Autodesk Fusion 360 part; units mm, degrees
(part 32 of 40)
  line L7913 (276.237, 134.1758) -> (276.3666, 134.08) construction
  line L7914 (276.3666, 134.08) -> (276.4958, 133.9832) construction
  line L7915 (276.4958, 133.9832) -> (276.6246, 133.8854) construction
  line L7916 (276.6246, 133.8854) -> (276.7529, 133.7868) construction
  line L7917 (276.7529, 133.7868) -> (276.8808, 133.6873) construction
  line L7918 (276.8808, 133.6873) -> (277.0082, 133.5869) construction
  line L7919 (277.0082, 133.5869) -> (277.1352, 133.4856) construction
  line L7920 (277.1352, 133.4856) -> (277.2618, 133.3834) construction
  line L7921 (277.2618, 133.3834) -> (277.388, 133.2804) construction
  line L7922 (277.388, 133.2804) -> (277.5137, 133.1765) construction
  line L7923 (277.5137, 133.1765) -> (277.639, 133.0717) construction
  line L7924 (277.639, 133.0717) -> (277.7638, 132.9662) construction
  line L7925 (277.7638, 132.9662) -> (277.8882, 132.8598) construction
  line L7926 (277.8882, 132.8598) -> (278.0122, 132.7526) construction
  line L7927 (278.0122, 132.7526) -> (278.1358, 132.6445) construction
  line L7928 (278.1358, 132.6445) -> (278.2589, 132.5357) construction
  line L7929 (278.2589, 132.5357) -> (278.3817, 132.4261) construction
  line L7930 (278.3817, 132.4261) -> (278.5039, 132.3158) construction
  line L7931 (278.5039, 132.3158) -> (278.6258, 132.2046) construction
  line L7932 (278.6258, 132.2046) -> (278.7472, 132.0927) construction
  line L7933 (278.7472, 132.0927) -> (278.8682, 131.98) construction
  line L7934 (278.8682, 131.98) -> (278.9888, 131.8665) construction
  line L7935 (278.9888, 131.8665) -> (279.1089, 131.7523) construction
  line L7936 (279.1089, 131.7523) -> (279.2286, 131.6374) construction
  line L7937 (279.2286, 131.6374) -> (279.3479, 131.5218) construction
  line L7938 (279.3479, 131.5218) -> (279.4667, 131.4054) construction
  line L7939 (279.4667, 131.4054) -> (279.5851, 131.2882) construction
  line L7940 (279.5851, 131.2882) -> (279.7031, 131.1704) construction
  line L7941 (279.7031, 131.1704) -> (279.8207, 131.0519) construction
  line L7942 (279.8207, 131.0519) -> (279.9378, 130.9326) construction
  line L7943 (279.9378, 130.9326) -> (280.0545, 130.8127) construction
  line L7944 (280.0545, 130.8127) -> (280.1708, 130.6921) construction
  line L7945 (280.1708, 130.6921) -> (280.2866, 130.5707) construction
  line L7946 (280.2866, 130.5707) -> (280.402, 130.4488) construction
  line L7947 (280.402, 130.4488) -> (280.517, 130.3261) construction
  line L7948 (280.517, 130.3261) -> (280.6087, 130.2274) construction
  line L7949 (280.6087, 130.2274) -> (280.6772, 130.1531) construction
  line L7950 (280.6772, 130.1531) -> (280.7228, 130.1034) construction
  line L7951 (280.7228, 130.1034) -> (280.7456, 130.0785) construction
  spline S106 degree 5 poles (187.9372, 206.0345) (187.9249, 206.0628) (187.9012, 206.1198) (187.868, 206.2062) (187.8281, 206.3229) (187.7842, 206.4711) (187.7447, 206.6208) (187.7079, 206.7714) (187.6725, 206.9226) (187.638, 207.0741) (187.6046, 207.226) (187.5726, 207.3783) (187.5424, 207.5312) (187.5144, 207.6848) (187.4885, 207.8391) (187.4646, 207.994) (187.4423, 208.1494) (187.4215, 208.3052) (187.4019, 208.4614) (187.3835, 208.6179) (187.3662, 208.7747) (187.3502, 208.9318) (187.3355, 209.0893) (187.3222, 209.2471) (187.3102, 209.4053) (187.2995, 209.5638) (187.29, 209.7226) (187.2816, 209.8817) (187.2743, 210.0411) (187.2682, 210.2007) (187.2631, 210.3605) (187.2591, 210.5206) (187.2563, 210.6809) (187.2544, 210.8415) (187.2537, 211.0023) (187.254, 211.1633) (187.2554, 211.3245) (187.2578, 211.4859) (187.2612, 211.6475) (187.2655, 211.8093) (187.2709, 211.9712) (187.2772, 212.1334) (187.2845, 212.2957) (187.2928, 212.4581) (187.302, 212.6207) (187.3121, 212.7835) (187.3232, 212.9464) (187.3353, 213.1095) (187.3482, 213.2727) (187.362, 213.436) (187.3768, 213.5995) (187.3924, 213.7631) (187.409, 213.9268) (187.4264, 214.0906) (187.4447, 214.2545) (187.4639, 214.4185) (187.484, 214.5826) (187.5049, 214.7468) (187.5266, 214.9111) (187.5492, 215.0755) (187.5727, 215.24) (187.597, 215.4046) (187.6222, 215.5692) (187.6481, 215.734) (187.6749, 215.8987) (187.7026, 216.0636) (187.731, 216.2285) (187.7602, 216.3935) (187.7903, 216.5585) (187.8212, 216.7236) (187.8528, 216.8887) (187.8788, 217.0208) (187.8986, 217.1199) (187.912, 217.186) (187.9188, 217.2191) knots 0 0 0 0 0 0 0.01428571 0.02857143 0.04285714 0.05714286 0.07142857 0.08571429 0.1 0.11428571 0.12857143 0.14285714 0.15714286 0.17142857 0.18571429 0.2 0.21428571 0.22857143 0.24285714 0.25714286 0.27142857 0.28571429 0.3 0.31428571 0.32857143 0.34285714 0.35714286 0.37142857 0.38571429 0.4 0.41428571 0.42857143 0.44285714 0.45714286 0.47142857 0.48571429 0.5 0.51428571 0.52857143 0.54285714 0.55714286 0.57142857 0.58571429 0.6 0.61428571 0.62857143 0.64285714 0.65714286 0.67142857 0.68571429 0.7 0.71428571 0.72857143 0.74285714 0.75714286 0.77142857 0.78571429 0.8 0.81428571 0.82857143 0.84285714 0.85714286 0.87142857 0.88571429 0.9 0.91428571 0.92857143 0.94285714 0.95714286 0.97142857 0.98571429 1 1 1 1 1 1
  line L7952 (187.9372, 206.0345) -> (187.9249, 206.0628) construction
  line L7953 (187.9249, 206.0628) -> (187.9012, 206.1198) construction
  line L7954 (187.9012, 206.1198) -> (187.868, 206.2062) construction
  line L7955 (187.868, 206.2062) -> (187.8281, 206.3229) construction
  line L7956 (187.8281, 206.3229) -> (187.7842, 206.4711) construction
  line L7957 (187.7842, 206.4711) -> (187.7447, 206.6208) construction
  line L7958 (187.7447, 206.6208) -> (187.7079, 206.7714) construction
  line L7959 (187.7079, 206.7714) -> (187.6725, 206.9226) construction
  line L7960 (187.6725, 206.9226) -> (187.638, 207.0741) construction
  line L7961 (187.638, 207.0741) -> (187.6046, 207.226) construction
  line L7962 (187.6046, 207.226) -> (187.5726, 207.3783) construction
  line L7963 (187.5726, 207.3783) -> (187.5424, 207.5312) construction
  line L7964 (187.5424, 207.5312) -> (187.5144, 207.6848) construction
  line L7965 (187.5144, 207.6848) -> (187.4885, 207.8391) construction
  line L7966 (187.4885, 207.8391) -> (187.4646, 207.994) construction
  line L7967 (187.4646, 207.994) -> (187.4423, 208.1494) construction
  line L7968 (187.4423, 208.1494) -> (187.4215, 208.3052) construction
  line L7969 (187.4215, 208.3052) -> (187.4019, 208.4614) construction
  line L7970 (187.4019, 208.4614) -> (187.3835, 208.6179) construction
  line L7971 (187.3835, 208.6179) -> (187.3662, 208.7747) construction
  line L7972 (187.3662, 208.7747) -> (187.3502, 208.9318) construction
  line L7973 (187.3502, 208.9318) -> (187.3355, 209.0893) construction
  line L7974 (187.3355, 209.0893) -> (187.3222, 209.2471) construction
  line L7975 (187.3222, 209.2471) -> (187.3102, 209.4053) construction
  line L7976 (187.3102, 209.4053) -> (187.2995, 209.5638) construction
  line L7977 (187.2995, 209.5638) -> (187.29, 209.7226) construction
  line L7978 (187.29, 209.7226) -> (187.2816, 209.8817) construction
  line L7979 (187.2816, 209.8817) -> (187.2743, 210.0411) construction
  line L7980 (187.2743, 210.0411) -> (187.2682, 210.2007) construction
  line L7981 (187.2682, 210.2007) -> (187.2631, 210.3605) construction
  line L7982 (187.2631, 210.3605) -> (187.2591, 210.5206) construction
  line L7983 (187.2591, 210.5206) -> (187.2563, 210.6809) construction
  line L7984 (187.2563, 210.6809) -> (187.2544, 210.8415) construction
  line L7985 (187.2544, 210.8415) -> (187.2537, 211.0023) construction
  line L7986 (187.2537, 211.0023) -> (187.254, 211.1633) construction
  line L7987 (187.254, 211.1633) -> (187.2554, 211.3245) construction
  line L7988 (187.2554, 211.3245) -> (187.2578, 211.4859) construction
  line L7989 (187.2578, 211.4859) -> (187.2612, 211.6475) construction
  line L7990 (187.2612, 211.6475) -> (187.2655, 211.8093) construction
  line L7991 (187.2655, 211.8093) -> (187.2709, 211.9712) construction
  line L7992 (187.2709, 211.9712) -> (187.2772, 212.1334) construction
  line L7993 (187.2772, 212.1334) -> (187.2845, 212.2957) construction
  line L7994 (187.2845, 212.2957) -> (187.2928, 212.4581) construction
  line L7995 (187.2928, 212.4581) -> (187.302, 212.6207) construction
  line L7996 (187.302, 212.6207) -> (187.3121, 212.7835) construction
  line L7997 (187.3121, 212.7835) -> (187.3232, 212.9464) construction
  line L7998 (187.3232, 212.9464) -> (187.3353, 213.1095) construction
  line L7999 (187.3353, 213.1095) -> (187.3482, 213.2727) construction
  line L8000 (187.3482, 213.2727) -> (187.362, 213.436) construction
  line L8001 (187.362, 213.436) -> (187.3768, 213.5995) construction
  line L8002 (187.3768, 213.5995) -> (187.3924, 213.7631) construction
  line L8003 (187.3924, 213.7631) -> (187.409, 213.9268) construction
  line L8004 (187.409, 213.9268) -> (187.4264, 214.0906) construction
  line L8005 (187.4264, 214.0906) -> (187.4447, 214.2545) construction
  line L8006 (187.4447, 214.2545) -> (187.4639, 214.4185) construction
  line L8007 (187.4639, 214.4185) -> (187.484, 214.5826) construction
  line L8008 (187.484, 214.5826) -> (187.5049, 214.7468) construction
  line L8009 (187.5049, 214.7468) -> (187.5266, 214.9111) construction
  line L8010 (187.5266, 214.9111) -> (187.5492, 215.0755) construction
  line L8011 (187.5492, 215.0755) -> (187.5727, 215.24) construction
  line L8012 (187.5727, 215.24) -> (187.597, 215.4046) construction
  line L8013 (187.597, 215.4046) -> (187.6222, 215.5692) construction
  line L8014 (187.6222, 215.5692) -> (187.6481, 215.734) construction
  line L8015 (187.6481, 215.734) -> (187.6749, 215.8987) construction
  line L8016 (187.6749, 215.8987) -> (187.7026, 216.0636) construction
  line L8017 (187.7026, 216.0636) -> (187.731, 216.2285) construction
  line L8018 (187.731, 216.2285) -> (187.7602, 216.3935) construction
  line L8019 (187.7602, 216.3935) -> (187.7903, 216.5585) construction
  line L8020 (187.7903, 216.5585) -> (187.8212, 216.7236) construction
  line L8021 (187.8212, 216.7236) -> (187.8528, 216.8887) construction
  line L8022 (187.8528, 216.8887) -> (187.8788, 217.0208) construction
  line L8023 (187.8788, 217.0208) -> (187.8986, 217.1199) construction
  line L8024 (187.8986, 217.1199) -> (187.912, 217.186) construction
  line L8025 (187.912, 217.186) -> (187.9188, 217.2191) construction
  arc A193 (161.7599, 177.5982) -> (160.1966, 174.5301) centre (212.132, 150) ccw
  arc A194 (232.0535, 81.3864) -> (236.3452, 82.7809) centre (212.132, 150) ccw
  arc A195 (155.1583, 142.7194) -> (155.697, 139.3184) centre (212.132, 150) ccw
  arc A196 (268.567, 139.3184) -> (269.1057, 142.7194) centre (212.132, 150) ccw
  spline S107 degree 5 poles (151.3635, 155.6951) (151.3327, 155.6979) (151.2711, 155.7029) (151.1787, 155.7078) (151.0554, 155.7097) (150.901, 155.7056) (150.7464, 155.6969) (150.5917, 155.6854) (150.437, 155.6723) (150.2822, 155.6583) (150.1275, 155.6431) (149.9727, 155.6265) (149.818, 155.608) (149.6632, 155.5871) (149.5085, 155.5641) (149.3538, 155.539) (149.1991, 155.5121) (149.0445, 155.4838) (148.8899, 155.4542) (148.7354, 155.4233) (148.5809, 155.3913) (148.4265, 155.3579) (148.2722, 155.3232) (148.118, 155.2871) (147.9638, 155.2497) (147.8098, 155.2109) (147.6558, 155.1709) (147.5019, 155.1297) (147.3481, 155.0873) (147.1944, 155.0439) (147.0408, 154.9993) (146.8873, 154.9536) (146.734, 154.9068) (146.5807, 154.8589) (146.4276, 154.8099) (146.2746, 154.7599) (146.1217, 154.7087) (145.9689, 154.6566) (145.8162, 154.6035) (145.6637, 154.5493) (145.5114, 154.4942) (145.3591, 154.438) (145.207, 154.381) (145.055, 154.3229) (144.9032, 154.2639) (144.7516, 154.2039) (144.6, 154.143) (144.4487, 154.0812) (144.2975, 154.0185) (144.1464, 153.9548) (143.9955, 153.8903) (143.8448, 153.8249) (143.6942, 153.7585) (143.5438, 153.6913) (143.3936, 153.6233) (143.2435, 153.5543) (143.0936, 153.4846) (142.9439, 153.4139) (142.7944, 153.3425) (142.645, 153.2701) (142.4958, 153.197) (142.3468, 153.123) (142.198, 153.0482) (142.0494, 152.9726) (141.9009, 152.8962) (141.7527, 152.819) (141.6046, 152.741) (141.4568, 152.6622) (141.3091, 152.5826) (141.1617, 152.5023) (141.0144, 152.4211) (140.8968, 152.3556) (140.8086, 152.3061) (140.7499, 152.2729) (140.7205, 152.2563) knots 0 0 0 0 0 0 0.01428571 0.02857143 0.04285714 0.05714286 0.07142857 0.08571429 0.1 0.11428571 0.12857143 0.14285714 0.15714286 0.17142857 0.18571429 0.2 0.21428571 0.22857143 0.24285714 0.25714286 0.27142857 0.28571429 0.3 0.31428571 0.32857143 0.34285714 0.35714286 0.37142857 0.38571429 0.4 0.41428571 0.42857143 0.44285714 0.45714286 0.47142857 0.48571429 0.5 0.51428571 0.52857143 0.54285714 0.55714286 0.57142857 0.58571429 0.6 0.61428571 0.62857143 0.64285714 0.65714286 0.67142857 0.68571429 0.7 0.71428571 0.72857143 0.74285714 0.75714286 0.77142857 0.78571429 0.8 0.81428571 0.82857143 0.84285714 0.85714286 0.87142857 0.88571429 0.9 0.91428571 0.92857143 0.94285714 0.95714286 0.97142857 0.98571429 1 1 1 1 1 1
  line L8026 (151.3635, 155.6951) -> (151.3327, 155.6979) construction
  line L8027 (151.3327, 155.6979) -> (151.2711, 155.7029) construction
  line L8028 (151.2711, 155.7029) -> (151.1787, 155.7078) construction
  line L8029 (151.1787, 155.7078) -> (151.0554, 155.7097) construction
  line L8030 (151.0554, 155.7097) -> (150.901, 155.7056) construction
  line L8031 (150.901, 155.7056) -> (150.7464, 155.6969) construction
  line L8032 (150.7464, 155.6969) -> (150.5917, 155.6854) construction
  line L8033 (150.5917, 155.6854) -> (150.437, 155.6723) construction
  line L8034 (150.437, 155.6723) -> (150.2822, 155.6583) construction
  line L8035 (150.2822, 155.6583) -> (150.1275, 155.6431) construction
  line L8036 (150.1275, 155.6431) -> (149.9727, 155.6265) construction
  line L8037 (149.9727, 155.6265) -> (149.818, 155.608) construction
  line L8038 (149.818, 155.608) -> (149.6632, 155.5871) construction
  line L8039 (149.6632, 155.5871) -> (149.5085, 155.5641) construction
  line L8040 (149.5085, 155.5641) -> (149.3538, 155.539) construction
  line L8041 (149.3538, 155.539) -> (149.1991, 155.5121) construction
  line L8042 (149.1991, 155.5121) -> (149.0445, 155.4838) construction
  line L8043 (149.0445, 155.4838) -> (148.8899, 155.4542) construction
  line L8044 (148.8899, 155.4542) -> (148.7354, 155.4233) construction
  line L8045 (148.7354, 155.4233) -> (148.5809, 155.3913) construction
  line L8046 (148.5809, 155.3913) -> (148.4265, 155.3579) construction
  line L8047 (148.4265, 155.3579) -> (148.2722, 155.3232) construction
  line L8048 (148.2722, 155.3232) -> (148.118, 155.2871) construction
  line L8049 (148.118, 155.2871) -> (147.9638, 155.2497) construction
  line L8050 (147.9638, 155.2497) -> (147.8098, 155.2109) construction
  line L8051 (147.8098, 155.2109) -> (147.6558, 155.1709) construction
  line L8052 (147.6558, 155.1709) -> (147.5019, 155.1297) construction
  line L8053 (147.5019, 155.1297) -> (147.3481, 155.0873) construction
  line L8054 (147.3481, 155.0873) -> (147.1944, 155.0439) construction
  line L8055 (147.1944, 155.0439) -> (147.0408, 154.9993) construction
  line L8056 (147.0408, 154.9993) -> (146.8873, 154.9536) construction
  line L8057 (146.8873, 154.9536) -> (146.734, 154.9068) construction
  line L8058 (146.734, 154.9068) -> (146.5807, 154.8589) construction
  line L8059 (146.5807, 154.8589) -> (146.4276, 154.8099) construction
  line L8060 (146.4276, 154.8099) -> (146.2746, 154.7599) construction
  line L8061 (146.2746, 154.7599) -> (146.1217, 154.7087) construction
  line L8062 (146.1217, 154.7087) -> (145.9689, 154.6566) construction
  line L8063 (145.9689, 154.6566) -> (145.8162, 154.6035) construction
  line L8064 (145.8162, 154.6035) -> (145.6637, 154.5493) construction
  line L8065 (145.6637, 154.5493) -> (145.5114, 154.4942) construction
  line L8066 (145.5114, 154.4942) -> (145.3591, 154.438) construction
  line L8067 (145.3591, 154.438) -> (145.207, 154.381) construction
  line L8068 (145.207, 154.381) -> (145.055, 154.3229) construction
  line L8069 (145.055, 154.3229) -> (144.9032, 154.2639) construction
  line L8070 (144.9032, 154.2639) -> (144.7516, 154.2039) construction
  line L8071 (144.7516, 154.2039) -> (144.6, 154.143) construction
  line L8072 (144.6, 154.143) -> (144.4487, 154.0812) construction
  line L8073 (144.4487, 154.0812) -> (144.2975, 154.0185) construction
  line L8074 (144.2975, 154.0185) -> (144.1464, 153.9548) construction
  line L8075 (144.1464, 153.9548) -> (143.9955, 153.8903) construction
  line L8076 (143.9955, 153.8903) -> (143.8448, 153.8249) construction
  line L8077 (143.8448, 153.8249) -> (143.6942, 153.7585) construction
  line L8078 (143.6942, 153.7585) -> (143.5438, 153.6913) construction
  line L8079 (143.5438, 153.6913) -> (143.3936, 153.6233) construction
  line L8080 (143.3936, 153.6233) -> (143.2435, 153.5543) construction
  line L8081 (143.2435, 153.5543) -> (143.0936, 153.4846) construction
  line L8082 (143.0936, 153.4846) -> (142.9439, 153.4139) construction
  line L8083 (142.9439, 153.4139) -> (142.7944, 153.3425) construction
  line L8084 (142.7944, 153.3425) -> (142.645, 153.2701) construction
  line L8085 (142.645, 153.2701) -> (142.4958, 153.197) construction
  line L8086 (142.4958, 153.197) -> (142.3468, 153.123) construction
  line L8087 (142.3468, 153.123) -> (142.198, 153.0482) construction
  line L8088 (142.198, 153.0482) -> (142.0494, 152.9726) construction
  line L8089 (142.0494, 152.9726) -> (141.9009, 152.8962) construction
  line L8090 (141.9009, 152.8962) -> (141.7527, 152.819) construction
  line L8091 (141.7527, 152.819) -> (141.6046, 152.741) construction
  line L8092 (141.6046, 152.741) -> (141.4568, 152.6622) construction
  line L8093 (141.4568, 152.6622) -> (141.3091, 152.5826) construction
  line L8094 (141.3091, 152.5826) -> (141.1617, 152.5023) construction
  line L8095 (141.1617, 152.5023) -> (141.0144, 152.4211) construction
  line L8096 (141.0144, 152.4211) -> (140.8968, 152.3556) construction
  line L8097 (140.8968, 152.3556) -> (140.8086, 152.3061) construction
  line L8098 (140.8086, 152.3061) -> (140.7499, 152.2729) construction
  line L8099 (140.7499, 152.2729) -> (140.7205, 152.2563) construction
  arc A197 (264.0674, 174.5301) -> (266.6686, 173.5481) centre (265.8758, 175.3842) ccw
  line L8100 (181.8522, 98.8934) -> (181.0205, 97.4897)
  line L8101 (181.8522, 201.1066) -> (181.0205, 202.5103)
  line L8102 (256.7226, 110.7517) -> (257.9473, 109.6737)
  line L8103 (172.8837, 105.4094) -> (171.8057, 104.1847)
  arc A198 (242.4118, 98.8934) -> (239.7302, 99.6279) centre (240.6912, 97.8739) ccw
  arc A199 (225.137, 92.0377) -> (222.8136, 93.565) centre (223.1855, 91.5999) ccw
  arc A200 (187.9188, 82.7809) -> (192.2105, 81.3864) centre (212.132, 150) ccw
  arc A201 (143.5184, 130.0785) -> (144.9129, 125.7868) centre (212.132, 150) ccw
  arc A202 (280.7456, 169.9215) -> (279.3511, 174.2132) centre (212.132, 150) ccw
  arc A203 (161.7599, 177.5982) -> (160.1966, 174.5301) centre (212.132, 150) ccw
  arc A204 (264.0674, 174.5301) -> (262.5041, 177.5982) centre (212.132, 150) ccw
  arc A205 (251.5104, 108.1868) -> (253.9452, 110.6216) centre (212.132, 150) ccw
  spline S108 degree 5 poles (225.4942, 90.4458) (225.501, 90.4157) (225.5153, 90.3556) (225.5391, 90.2662) (225.5755, 90.1483) (225.6271, 90.0027) (225.6831, 89.8584) (225.7419, 89.7148) (225.8021, 89.5717) (225.8633, 89.4289) (225.9255, 89.2864) (225.9891, 89.1443) (226.0546, 89.0029) (226.1222, 88.8621) (226.192, 88.7221) (226.2636, 88.5827) (226.337, 88.4439) (226.4117, 88.3056) (226.4877, 88.1678) (226.5647, 88.0303) (226.6429, 87.8933) (226.7224, 87.7568) (226.8031, 87.6208) (226.885, 87.4852) (226.9683, 87.3502) (227.0528, 87.2157) (227.1384, 87.0816) (227.2252, 86.948) (227.313, 86.8148) (227.4018, 86.682) (227.4917, 86.5497) (227.5826, 86.4179) (227.6745, 86.2865) (227.7674, 86.1555) (227.8613, 86.025) (227.9562, 85.895) (228.052, 85.7654) (228.1488, 85.6362) (228.2466, 85.5074) (228.3452, 85.3791) (228.4447, 85.2512) (228.5451, 85.1238) (228.6464, 84.9968) (228.7486, 84.8702) (228.8516, 84.744) (228.9555, 84.6183) (229.0603, 84.493) (229.1658, 84.3682) (229.2722, 84.2438) (229.3794, 84.1198) (229.4875, 83.9962) (229.5963, 83.8731) (229.7059, 83.7503) (229.8162, 83.6281) (229.9274, 83.5062) (230.0393, 83.3848) (230.152, 83.2638) (230.2655, 83.1432) (230.3797, 83.0231) (230.4946, 82.9034) (230.6102, 82.7841) (230.7266, 82.6653) (230.8438, 82.5469) (230.9616, 82.4289) (231.0801, 82.3113) (231.1994, 82.1942) (231.3193, 82.0775) (231.4399, 81.9612) (231.5613, 81.8454) (231.6832, 81.73) (231.8059, 81.615) (231.9046, 81.5233) (231.9789, 81.4548) (232.0286, 81.4092) (232.0535, 81.3864) knots 0 0 0 0 0 0 0.01428571 0.02857143 0.04285714 0.05714286 0.07142857 0.08571429 0.1 0.11428571 0.12857143 0.14285714 0.15714286 0.17142857 0.18571429 0.2 0.21428571 0.22857143 0.24285714 0.25714286 0.27142857 0.28571429 0.3 0.31428571 0.32857143 0.34285714 0.35714286 0.37142857 0.38571429 0.4 0.41428571 0.42857143 0.44285714 0.45714286 0.47142857 0.48571429 0.5 0.51428571 0.52857143 0.54285714 0.55714286 0.57142857 0.58571429 0.6 0.61428571 0.62857143 0.64285714 0.65714286 0.67142857 0.68571429 0.7 0.71428571 0.72857143 0.74285714 0.75714286 0.77142857 0.78571429 0.8 0.81428571 0.82857143 0.84285714 0.85714286 0.87142857 0.88571429 0.9 0.91428571 0.92857143 0.94285714 0.95714286 0.97142857 0.98571429 1 1 1 1 1 1
  line L8104 (225.4942, 90.4458) -> (225.501, 90.4157) construction
  line L8105 (225.501, 90.4157) -> (225.5153, 90.3556) construction
  line L8106 (225.5153, 90.3556) -> (225.5391, 90.2662) construction
  line L8107 (225.5391, 90.2662) -> (225.5755, 90.1483) construction
  line L8108 (225.5755, 90.1483) -> (225.6271, 90.0027) construction
  line L8109 (225.6271, 90.0027) -> (225.6831, 89.8584) construction
  line L8110 (225.6831, 89.8584) -> (225.7419, 89.7148) construction
  line L8111 (225.7419, 89.7148) -> (225.8021, 89.5717) construction
  line L8112 (225.8021, 89.5717) -> (225.8633, 89.4289) construction
  line L8113 (225.8633, 89.4289) -> (225.9255, 89.2864) construction
  line L8114 (225.9255, 89.2864) -> (225.9891, 89.1443) construction
  line L8115 (225.9891, 89.1443) -> (226.0546, 89.0029) construction
  line L8116 (226.0546, 89.0029) -> (226.1222, 88.8621) construction
  line L8117 (226.1222, 88.8621) -> (226.192, 88.7221) construction
  line L8118 (226.192, 88.7221) -> (226.2636, 88.5827) construction
  line L8119 (226.2636, 88.5827) -> (226.337, 88.4439) construction
  line L8120 (226.337, 88.4439) -> (226.4117, 88.3056) construction
  line L8121 (226.4117, 88.3056) -> (226.4877, 88.1678) construction
  line L8122 (226.4877, 88.1678) -> (226.5647, 88.0303) construction
  line L8123 (226.5647, 88.0303) -> (226.6429, 87.8933) construction
  line L8124 (226.6429, 87.8933) -> (226.7224, 87.7568) construction
  line L8125 (226.7224, 87.7568) -> (226.8031, 87.6208) construction
  line L8126 (226.8031, 87.6208) -> (226.885, 87.4852) construction
  line L8127 (226.885, 87.4852) -> (226.9683, 87.3502) construction
  line L8128 (226.9683, 87.3502) -> (227.0528, 87.2157) construction
  line L8129 (227.0528, 87.2157) -> (227.1384, 87.0816) construction
  line L8130 (227.1384, 87.0816) -> (227.2252, 86.948) construction
  line L8131 (227.2252, 86.948) -> (227.313, 86.8148) construction
  line L8132 (227.313, 86.8148) -> (227.4018, 86.682) construction
  line L8133 (227.4018, 86.682) -> (227.4917, 86.5497) construction
  line L8134 (227.4917, 86.5497) -> (227.5826, 86.4179) construction
  line L8135 (227.5826, 86.4179) -> (227.6745, 86.2865) construction
  line L8136 (227.6745, 86.2865) -> (227.7674, 86.1555) construction
  line L8137 (227.7674, 86.1555) -> (227.8613, 86.025) construction
  line L8138 (227.8613, 86.025) -> (227.9562, 85.895) construction
  line L8139 (227.9562, 85.895) -> (228.052, 85.7654) construction
  line L8140 (228.052, 85.7654) -> (228.1488, 85.6362) construction
  line L8141 (228.1488, 85.6362) -> (228.2466, 85.5074) construction
  line L8142 (228.2466, 85.5074) -> (228.3452, 85.3791) construction
  line L8143 (228.3452, 85.3791) -> (228.4447, 85.2512) construction
  line L8144 (228.4447, 85.2512) -> (228.5451, 85.1238) construction
  line L8145 (228.5451, 85.1238) -> (228.6464, 84.9968) construction
  line L8146 (228.6464, 84.9968) -> (228.7486, 84.8702) construction
  line L8147 (228.7486, 84.8702) -> (228.8516, 84.744) construction
  line L8148 (228.8516, 84.744) -> (228.9555, 84.6183) construction
  line L8149 (228.9555, 84.6183) -> (229.0603, 84.493) construction
  line L8150 (229.0603, 84.493) -> (229.1658, 84.3682) construction
  line L8151 (229.1658, 84.3682) -> (229.2722, 84.2438) construction
  line L8152 (229.2722, 84.2438) -> (229.3794, 84.1198) construction
  line L8153 (229.3794, 84.1198) -> (229.4875, 83.9962) construction
  line L8154 (229.4875, 83.9962) -> (229.5963, 83.8731) construction
  line L8155 (229.5963, 83.8731) -> (229.7059, 83.7503) construction
  line L8156 (229.7059, 83.7503) -> (229.8162, 83.6281) construction
  line L8157 (229.8162, 83.6281) -> (229.9274, 83.5062) construction
  line L8158 (229.9274, 83.5062) -> (230.0393, 83.3848) construction
  line L8159 (230.0393, 83.3848) -> (230.152, 83.2638) construction
  line L8160 (230.152, 83.2638) -> (230.2655, 83.1432) construction
  line L8161 (230.2655, 83.1432) -> (230.3797, 83.0231) construction
  line L8162 (230.3797, 83.0231) -> (230.4946, 82.9034) construction
  line L8163 (230.4946, 82.9034) -> (230.6102, 82.7841) construction
  line L8164 (230.6102, 82.7841) -> (230.7266, 82.6653) construction
  line L8165 (230.7266, 82.6653) -> (230.8438, 82.5469) construction
  line L8166 (230.8438, 82.5469) -> (230.9616, 82.4289) construction
  line L8167 (230.9616, 82.4289) -> (231.0801, 82.3113) construction
  line L8168 (231.0801, 82.3113) -> (231.1994, 82.1942) construction
  line L8169 (231.1994, 82.1942) -> (231.3193, 82.0775) construction
  line L8170 (231.3193, 82.0775) -> (231.4399, 81.9612) construction
  line L8171 (231.4399, 81.9612) -> (231.5613, 81.8454) construction
  line L8172 (231.5613, 81.8454) -> (231.6832, 81.73) construction
  line L8173 (231.6832, 81.73) -> (231.8059, 81.615) construction
  line L8174 (231.8059, 81.615) -> (231.9046, 81.5233) construction
  line L8175 (231.9046, 81.5233) -> (231.9789, 81.4548) construction
  line L8176 (231.9789, 81.4548) -> (232.0286, 81.4092) construction
  line L8177 (232.0286, 81.4092) -> (232.0535, 81.3864) construction
  spline S109 degree 5 poles (252.4583, 104.1847) (252.4787, 104.1615) (252.5188, 104.1146) (252.5771, 104.0427) (252.6512, 103.944) (252.7386, 103.8167) (252.8224, 103.6865) (252.904, 103.5546) (252.9844, 103.4218) (253.064, 103.2883) (253.1427, 103.1542) (253.2203, 103.0193) (253.2962, 102.8832) (253.3703, 102.7457) (253.4426, 102.607) (253.5133, 102.4671) (253.5824, 102.3262) (253.6504, 102.1844) (253.7173, 102.0419) (253.7832, 101.8988) (253.848, 101.755) (253.9118, 101.6105) (253.9744, 101.4653) (254.0359, 101.3193) (254.0962, 101.1726) (254.1554, 101.0251) (254.2135, 100.877) (254.2706, 100.7283) (254.3267, 100.579) (254.3819, 100.4291) (254.4361, 100.2786) (254.4894, 100.1276) (254.5417, 99.976) (254.593, 99.8239) (254.6434, 99.6712) (254.6928, 99.518) (254.7414, 99.3642) (254.789, 99.21) (254.8357, 99.0553) (254.8815, 98.9001) (254.9265, 98.7444) (254.9706, 98.5882) (255.0138, 98.4316) (255.0561, 98.2745) (255.0976, 98.117) (255.1383, 97.9591) (255.1781, 97.8007) (255.217, 97.6419) (255.2551, 97.4827) (255.2924, 97.3231) (255.3289, 97.1631) (255.3646, 97.0027) (255.3994, 96.8419) (255.4335, 96.6807) (255.4667, 96.5191) (255.4992, 96.3572) (255.5308, 96.1949) (255.5617, 96.0323) (255.5917, 95.8693) (255.621, 95.706) (255.6495, 95.5423) (255.6773, 95.3783) (255.7043, 95.2139) (255.7304, 95.0492) (255.7559, 94.8842) (255.7806, 94.7189) (255.8045, 94.5533) (255.8276, 94.3874) (255.85, 94.2211) (255.8717, 94.0546) (255.8926, 93.8878) (255.9087, 93.7541) (255.9205, 93.6537) (255.9282, 93.5867) (255.932, 93.5531) knots 0 0 0 0 0 0 0.01428571 0.02857143 0.04285714 0.05714286 0.07142857 0.08571429 0.1 0.11428571 0.12857143 0.14285714 0.15714286 0.17142857 0.18571429 0.2 0.21428571 0.22857143 0.24285714 0.25714286 0.27142857 0.28571429 0.3 0.31428571 0.32857143 0.34285714 0.35714286 0.37142857 0.38571429 0.4 0.41428571 0.42857143 0.44285714 0.45714286 0.47142857 0.48571429 0.5 0.51428571 0.52857143 0.54285714 0.55714286 0.57142857 0.58571429 0.6 0.61428571 0.62857143 0.64285714 0.65714286 0.67142857 0.68571429 0.7 0.71428571 0.72857143 0.74285714 0.75714286 0.77142857 0.78571429 0.8 0.81428571 0.82857143 0.84285714 0.85714286 0.87142857 0.88571429 0.9 0.91428571 0.92857143 0.94285714 0.95714286 0.97142857 0.98571429 1 1 1 1 1 1
  line L8178 (252.4583, 104.1847) -> (252.4787, 104.1615) construction
  line L8179 (252.4787, 104.1615) -> (252.5188, 104.1146) construction
  line L8180 (252.5188, 104.1146) -> (252.5771, 104.0427) construction
  line L8181 (252.5771, 104.0427) -> (252.6512, 103.944) construction
  line L8182 (252.6512, 103.944) -> (252.7386, 103.8167) construction
  line L8183 (252.7386, 103.8167) -> (252.8224, 103.6865) construction
  line L8184 (252.8224, 103.6865) -> (252.904, 103.5546) construction
  line L8185 (252.904, 103.5546) -> (252.9844, 103.4218) construction
  line L8186 (252.9844, 103.4218) -> (253.064, 103.2883) construction
  line L8187 (253.064, 103.2883) -> (253.1427, 103.1542) construction
  line L8188 (253.1427, 103.1542) -> (253.2203, 103.0193) construction
  line L8189 (253.2203, 103.0193) -> (253.2962, 102.8832) construction
  line L8190 (253.2962, 102.8832) -> (253.3703, 102.7457) construction
  line L8191 (253.3703, 102.7457) -> (253.4426, 102.607) construction
  line L8192 (253.4426, 102.607) -> (253.5133, 102.4671) construction
  line L8193 (253.5133, 102.4671) -> (253.5824, 102.3262) construction
  line L8194 (253.5824, 102.3262) -> (253.6504, 102.1844) construction
  line L8195 (253.6504, 102.1844) -> (253.7173, 102.0419) construction
  line L8196 (253.7173, 102.0419) -> (253.7832, 101.8988) construction
  line L8197 (253.7832, 101.8988) -> (253.848, 101.755) construction
  line L8198 (253.848, 101.755) -> (253.9118, 101.6105) construction
  line L8199 (253.9118, 101.6105) -> (253.9744, 101.4653) construction
  line L8200 (253.9744, 101.4653) -> (254.0359, 101.3193) construction
  line L8201 (254.0359, 101.3193) -> (254.0962, 101.1726) construction
  line L8202 (254.0962, 101.1726) -> (254.1554, 101.0251) construction
  line L8203 (254.1554, 101.0251) -> (254.2135, 100.877) construction
  line L8204 (254.2135, 100.877) -> (254.2706, 100.7283) construction
  line L8205 (254.2706, 100.7283) -> (254.3267, 100.579) construction
  line L8206 (254.3267, 100.579) -> (254.3819, 100.4291) construction
  line L8207 (254.3819, 100.4291) -> (254.4361, 100.2786) construction
  line L8208 (254.4361, 100.2786) -> (254.4894, 100.1276) construction
  line L8209 (254.4894, 100.1276) -> (254.5417, 99.976) construction
  line L8210 (254.5417, 99.976) -> (254.593, 99.8239) construction
  line L8211 (254.593, 99.8239) -> (254.6434, 99.6712) construction
  line L8212 (254.6434, 99.6712) -> (254.6928, 99.518) construction
  line L8213 (254.6928, 99.518) -> (254.7414, 99.3642) construction
  line L8214 (254.7414, 99.3642) -> (254.789, 99.21) construction
  line L8215 (254.789, 99.21) -> (254.8357, 99.0553) construction
  line L8216 (254.8357, 99.0553) -> (254.8815, 98.9001) construction
  line L8217 (254.8815, 98.9001) -> (254.9265, 98.7444) construction
  line L8218 (254.9265, 98.7444) -> (254.9706, 98.5882) construction
  line L8219 (254.9706, 98.5882) -> (255.0138, 98.4316) construction
  line L8220 (255.0138, 98.4316) -> (255.0561, 98.2745) construction
  line L8221 (255.0561, 98.2745) -> (255.0976, 98.117) construction
  line L8222 (255.0976, 98.117) -> (255.1383, 97.9591) construction
  line L8223 (255.1383, 97.9591) -> (255.1781, 97.8007) construction
  line L8224 (255.1781, 97.8007) -> (255.217, 97.6419) construction
  line L8225 (255.217, 97.6419) -> (255.2551, 97.4827) construction
  line L8226 (255.2551, 97.4827) -> (255.2924, 97.3231) construction
  line L8227 (255.2924, 97.3231) -> (255.3289, 97.1631) construction
  line L8228 (255.3289, 97.1631) -> (255.3646, 97.0027) construction
  line L8229 (255.3646, 97.0027) -> (255.3994, 96.8419) construction
  line L8230 (255.3994, 96.8419) -> (255.4335, 96.6807) construction
  line L8231 (255.4335, 96.6807) -> (255.4667, 96.5191) construction
  line L8232 (255.4667, 96.5191) -> (255.4992, 96.3572) construction
  line L8233 (255.4992, 96.3572) -> (255.5308, 96.1949) construction
  line L8234 (255.5308, 96.1949) -> (255.5617, 96.0323) construction
  line L8235 (255.5617, 96.0323) -> (255.5917, 95.8693) construction
  line L8236 (255.5917, 95.8693) -> (255.621, 95.706) construction
  line L8237 (255.621, 95.706) -> (255.6495, 95.5423) construction
  line L8238 (255.6495, 95.5423) -> (255.6773, 95.3783) construction
  line L8239 (255.6773, 95.3783) -> (255.7043, 95.2139) construction
  line L8240 (255.7043, 95.2139) -> (255.7304, 95.0492) construction
  line L8241 (255.7304, 95.0492) -> (255.7559, 94.8842) construction
  line L8242 (255.7559, 94.8842) -> (255.7806, 94.7189) construction
  line L8243 (255.7806, 94.7189) -> (255.8045, 94.5533) construction
  line L8244 (255.8045, 94.5533) -> (255.8276, 94.3874) construction
  line L8245 (255.8276, 94.3874) -> (255.85, 94.2211) construction
  line L8246 (255.85, 94.2211) -> (255.8717, 94.0546) construction
  line L8247 (255.8717, 94.0546) -> (255.8926, 93.8878) construction
  line L8248 (255.8926, 93.8878) -> (255.9087, 93.7541) construction
  line L8249 (255.9087, 93.7541) -> (255.9205, 93.6537) construction
  line L8250 (255.9205, 93.6537) -> (255.9282, 93.5867) construction
  line L8251 (255.9282, 93.5867) -> (255.932, 93.5531) construction
  arc A206 (236.6621, 98.0646) -> (239.7302, 99.6279) centre (212.132, 150) ccw
  arc A207 (255.932, 206.4469) -> (252.2812, 209.0993) centre (212.132, 150) ccw
  spline S110 degree 5 poles (151.3635, 144.3049) (151.3327, 144.3021) (151.2711, 144.2971) (151.1787, 144.2922) (151.0554, 144.2903) (150.901, 144.2944) (150.7464, 144.3031) (150.5917, 144.3146) (150.437, 144.3277) (150.2822, 144.3417) (150.1275, 144.3569) (149.9727, 144.3735) (149.818, 144.392) (149.6632, 144.4129) (149.5085, 144.4359) (149.3538, 144.461) (149.1991, 144.4879) (149.0445, 144.5162) (148.8899, 144.5458) (148.7354, 144.5767) (148.5809, 144.6087) (148.4265, 144.6421) (148.2722, 144.6768) (148.118, 144.7129) (147.9638, 144.7503) (147.8098, 144.7891) (147.6558, 144.8291) (147.5019, 144.8703) (147.3481, 144.9127) (147.1944, 144.9561) (147.0408, 145.0007) (146.8873, 145.0464) (146.734, 145.0932) (146.5807, 145.1411) (146.4276, 145.1901) (146.2746, 145.2401) (146.1217, 145.2913) (145.9689, 145.3434) (145.8162, 145.3965) (145.6637, 145.4507) (145.5114, 145.5058) (145.3591, 145.562) (145.207, 145.619) (145.055, 145.6771) (144.9032, 145.7361) (144.7516, 145.7961) (144.6, 145.857) (144.4487, 145.9188) (144.2975, 145.9815) (144.1464, 146.0452) (143.9955, 146.1097) (143.8448, 146.1751) (143.6942, 146.2415) (143.5438, 146.3087) (143.3936, 146.3767) (143.2435, 146.4457) (143.0936, 146.5154) (142.9439, 146.5861) (142.7944, 146.6575) (142.645, 146.7299) (142.4958, 146.803) (142.3468, 146.877) (142.198, 146.9518) (142.0494, 147.0274) (141.9009, 147.1038) (141.7527, 147.181) (141.6046, 147.259) (141.4568, 147.3378) (141.3091, 147.4174) (141.1617, 147.4977) (141.0144, 147.5789) (140.8968, 147.6444) (140.8086, 147.6939) (140.7499, 147.7271) (140.7205, 147.7437) knots 0 0 0 0 0 0 0.01428571 0.02857143 0.04285714 0.05714286 0.07142857 0.08571429 0.1 0.11428571 0.12857143 0.14285714 0.15714286 0.17142857 0.18571429 0.2 0.21428571 0.22857143 0.24285714 0.25714286 0.27142857 0.28571429 0.3 0.31428571 0.32857143 0.34285714 0.35714286 0.37142857 0.38571429 0.4 0.41428571 0.42857143 0.44285714 0.45714286 0.47142857 0.48571429 0.5 0.51428571 0.52857143 0.54285714 0.55714286 0.57142857 0.58571429 0.6 0.61428571 0.62857143 0.64285714 0.65714286 0.67142857 0.68571429 0.7 0.71428571 0.72857143 0.74285714 0.75714286 0.77142857 0.78571429 0.8 0.81428571 0.82857143 0.84285714 0.85714286 0.87142857 0.88571429 0.9 0.91428571 0.92857143 0.94285714 0.95714286 0.97142857 0.98571429 1 1 1 1 1 1
  line L8252 (151.3635, 144.3049) -> (151.3327, 144.3021) construction
  line L8253 (151.3327, 144.3021) -> (151.2711, 144.2971) construction
  line L8254 (151.2711, 144.2971) -> (151.1787, 144.2922) construction
  line L8255 (151.1787, 144.2922) -> (151.0554, 144.2903) construction
  line L8256 (151.0554, 144.2903) -> (150.901, 144.2944) construction
  line L8257 (150.901, 144.2944) -> (150.7464, 144.3031) construction
  line L8258 (150.7464, 144.3031) -> (150.5917, 144.3146) construction
  line L8259 (150.5917, 144.3146) -> (150.437, 144.3277) construction
  line L8260 (150.437, 144.3277) -> (150.2822, 144.3417) construction
  line L8261 (150.2822, 144.3417) -> (150.1275, 144.3569) construction
  line L8262 (150.1275, 144.3569) -> (149.9727, 144.3735) construction
  line L8263 (149.9727, 144.3735) -> (149.818, 144.392) construction
  line L8264 (149.818, 144.392) -> (149.6632, 144.4129) construction
  line L8265 (149.6632, 144.4129) -> (149.5085, 144.4359) construction
  line L8266 (149.5085, 144.4359) -> (149.3538, 144.461) construction
  line L8267 (149.3538, 144.461) -> (149.1991, 144.4879) construction
  line L8268 (149.1991, 144.4879) -> (149.0445, 144.5162) construction
  line L8269 (149.0445, 144.5162) -> (148.8899, 144.5458) construction
  line L8270 (148.8899, 144.5458) -> (148.7354, 144.5767) construction
  line L8271 (148.7354, 144.5767) -> (148.5809, 144.6087) construction
  line L8272 (148.5809, 144.6087) -> (148.4265, 144.6421) construction
  line L8273 (148.4265, 144.6421) -> (148.2722, 144.6768) construction
  line L8274 (148.2722, 144.6768) -> (148.118, 144.7129) construction
  line L8275 (148.118, 144.7129) -> (147.9638, 144.7503) construction
  line L8276 (147.9638, 144.7503) -> (147.8098, 144.7891) construction
  line L8277 (147.8098, 144.7891) -> (147.6558, 144.8291) construction
  line L8278 (147.6558, 144.8291) -> (147.5019, 144.8703) construction
  line L8279 (147.5019, 144.8703) -> (147.3481, 144.9127) construction
  line L8280 (147.3481, 144.9127) -> (147.1944, 144.9561) construction
  line L8281 (147.1944, 144.9561) -> (147.0408, 145.0007) construction
  line L8282 (147.0408, 145.0007) -> (146.8873, 145.0464) construction
  line L8283 (146.8873, 145.0464) -> (146.734, 145.0932) construction
  line L8284 (146.734, 145.0932) -> (146.5807, 145.1411) construction
  line L8285 (146.5807, 145.1411) -> (146.4276, 145.1901) construction
  line L8286 (146.4276, 145.1901) -> (146.2746, 145.2401) construction
  line L8287 (146.2746, 145.2401) -> (146.1217, 145.2913) construction
  line L8288 (146.1217, 145.2913) -> (145.9689, 145.3434) construction
  line L8289 (145.9689, 145.3434) -> (145.8162, 145.3965) construction
  line L8290 (145.8162, 145.3965) -> (145.6637, 145.4507) construction
  line L8291 (145.6637, 145.4507) -> (145.5114, 145.5058) construction
  line L8292 (145.5114, 145.5058) -> (145.3591, 145.562) construction
  line L8293 (145.3591, 145.562) -> (145.207, 145.619) construction
  line L8294 (145.207, 145.619) -> (145.055, 145.6771) construction
  line L8295 (145.055, 145.6771) -> (144.9032, 145.7361) construction
  line L8296 (144.9032, 145.7361) -> (144.7516, 145.7961) construction
  line L8297 (144.7516, 145.7961) -> (144.6, 145.857) construction
  line L8298 (144.6, 145.857) -> (144.4487, 145.9188) construction
  line L8299 (144.4487, 145.9188) -> (144.2975, 145.9815) construction
  line L8300 (144.2975, 145.9815) -> (144.1464, 146.0452) construction
  line L8301 (144.1464, 146.0452) -> (143.9955, 146.1097) construction
  line L8302 (143.9955, 146.1097) -> (143.8448, 146.1751) construction
  line L8303 (143.8448, 146.1751) -> (143.6942, 146.2415) construction
  line L8304 (143.6942, 146.2415) -> (143.5438, 146.3087) construction
  line L8305 (143.5438, 146.3087) -> (143.3936, 146.3767) construction
  line L8306 (143.3936, 146.3767) -> (143.2435, 146.4457) construction
  line L8307 (143.2435, 146.4457) -> (143.0936, 146.5154) construction
  line L8308 (143.0936, 146.5154) -> (142.9439, 146.5861) construction
  line L8309 (142.9439, 146.5861) -> (142.7944, 146.6575) construction
  line L8310 (142.7944, 146.6575) -> (142.645, 146.7299) construction
  line L8311 (142.645, 146.7299) -> (142.4958, 146.803) construction
  line L8312 (142.4958, 146.803) -> (142.3468, 146.877) construction
  line L8313 (142.3468, 146.877) -> (142.198, 146.9518) construction
  line L8314 (142.198, 146.9518) -> (142.0494, 147.0274) construction
  line L8315 (142.0494, 147.0274) -> (141.9009, 147.1038) construction
  line L8316 (141.9009, 147.1038) -> (141.7527, 147.181) construction
  line L8317 (141.7527, 147.181) -> (141.6046, 147.259) construction
  line L8318 (141.6046, 147.259) -> (141.4568, 147.3378) construction
  line L8319 (141.4568, 147.3378) -> (141.3091, 147.4174) construction
  line L8320 (141.3091, 147.4174) -> (141.1617, 147.4977) construction
  line L8321 (141.1617, 147.4977) -> (141.0144, 147.5789) construction
  line L8322 (141.0144, 147.5789) -> (140.8968, 147.6444) construction
  line L8323 (140.8968, 147.6444) -> (140.8086, 147.6939) construction
  line L8324 (140.8086, 147.6939) -> (140.7499, 147.7271) construction
  line L8325 (140.7499, 147.7271) -> (140.7205, 147.7437) construction
  arc A208 (201.4504, 93.565) -> (199.127, 92.0377) centre (201.0785, 91.5999) ccw
  spline S111 degree 5 poles (206.4369, 210.7685) (206.4341, 210.7993) (206.4291, 210.8609) (206.4242, 210.9533) (206.4223, 211.0766) (206.4264, 211.231) (206.4351, 211.3856) (206.4466, 211.5403) (206.4597, 211.695) (206.4737, 211.8498) (206.4889, 212.0045) (206.5055, 212.1593) (206.524, 212.314) (206.5449, 212.4688) (206.5679, 212.6235) (206.593, 212.7782) (206.6199, 212.9329) (206.6482, 213.0875) (206.6778, 213.2421) (206.7087, 213.3966) (206.7407, 213.5511) (206.7741, 213.7055) (206.8088, 213.8598) (206.8449, 214.014) (206.8823, 214.1682) (206.9211, 214.3222) (206.9611, 214.4762) (207.0023, 214.6301) (207.0447, 214.7839) (207.0881, 214.9376) (207.1327, 215.0912) (207.1784, 215.2447) (207.2252, 215.398) (207.2731, 215.5513) (207.3221, 215.7044) (207.3721, 215.8574) (207.4233, 216.0103) (207.4754, 216.1631) (207.5285, 216.3158) (207.5827, 216.4683) (207.6378, 216.6206) (207.694, 216.7729) (207.751, 216.925) (207.8091, 217.077) (207.8681, 217.2288) (207.9281, 217.3804) (207.989, 217.532) (208.0508, 217.6833) (208.1135, 217.8345) (208.1772, 217.9856) (208.2417, 218.1365) (208.3071, 218.2872) (208.3735, 218.4378) (208.4407, 218.5882) (208.5087, 218.7384) (208.5777, 218.8885) (208.6474, 219.0384) (208.7181, 219.1881) (208.7895, 219.3376) (208.8619, 219.487) (208.935, 219.6362) (209.009, 219.7852) (209.0838, 219.934) (209.1594, 220.0826) (209.2358, 220.2311) (209.313, 220.3793) (209.391, 220.5274) (209.4698, 220.6752) (209.5494, 220.8229) (209.6297, 220.9703) (209.7109, 221.1176) (209.7764, 221.2352) (209.8259, 221.3234) (209.8591, 221.3821) (209.8757, 221.4115) knots 0 0 0 0 0 0 0.01428571 0.02857143 0.04285714 0.05714286 0.07142857 0.08571429 0.1 0.11428571 0.12857143 0.14285714 0.15714286 0.17142857 0.18571429 0.2 0.21428571 0.22857143 0.24285714 0.25714286 0.27142857 0.28571429 0.3 0.31428571 0.32857143 0.34285714 0.35714286 0.37142857 0.38571429 0.4 0.41428571 0.42857143 0.44285714 0.45714286 0.47142857 0.48571429 0.5 0.51428571 0.52857143 0.54285714 0.55714286 0.57142857 0.58571429 0.6 0.61428571 0.62857143 0.64285714 0.65714286 0.67142857 0.68571429 0.7 0.71428571 0.72857143 0.74285714 0.75714286 0.77142857 0.78571429 0.8 0.81428571 0.82857143 0.84285714 0.85714286 0.87142857 0.88571429 0.9 0.91428571 0.92857143 0.94285714 0.95714286 0.97142857 0.98571429 1 1 1 1 1 1
  line L8326 (206.4369, 210.7685) -> (206.4341, 210.7993) construction
  line L8327 (206.4341, 210.7993) -> (206.4291, 210.8609) construction
  line L8328 (206.4291, 210.8609) -> (206.4242, 210.9533) construction
  line L8329 (206.4242, 210.9533) -> (206.4223, 211.0766) construction
  line L8330 (206.4223, 211.0766) -> (206.4264, 211.231) construction
  line L8331 (206.4264, 211.231) -> (206.4351, 211.3856) construction
  line L8332 (206.4351, 211.3856) -> (206.4466, 211.5403) construction
  line L8333 (206.4466, 211.5403) -> (206.4597, 211.695) construction
  line L8334 (206.4597, 211.695) -> (206.4737, 211.8498) construction
  line L8335 (206.4737, 211.8498) -> (206.4889, 212.0045) construction
  line L8336 (206.4889, 212.0045) -> (206.5055, 212.1593) construction
  line L8337 (206.5055, 212.1593) -> (206.524, 212.314) construction
  line L8338 (206.524, 212.314) -> (206.5449, 212.4688) construction
  line L8339 (206.5449, 212.4688) -> (206.5679, 212.6235) construction
  line L8340 (206.5679, 212.6235) -> (206.593, 212.7782) construction
  line L8341 (206.593, 212.7782) -> (206.6199, 212.9329) construction
  line L8342 (206.6199, 212.9329) -> (206.6482, 213.0875) construction
  line L8343 (206.6482, 213.0875) -> (206.6778, 213.2421) construction
  line L8344 (206.6778, 213.2421) -> (206.7087, 213.3966) construction
  line L8345 (206.7087, 213.3966) -> (206.7407, 213.5511) construction
  line L8346 (206.7407, 213.5511) -> (206.7741, 213.7055) construction
  line L8347 (206.7741, 213.7055) -> (206.8088, 213.8598) construction
  line L8348 (206.8088, 213.8598) -> (206.8449, 214.014) construction
  line L8349 (206.8449, 214.014) -> (206.8823, 214.1682) construction
  line L8350 (206.8823, 214.1682) -> (206.9211, 214.3222) construction
  line L8351 (206.9211, 214.3222) -> (206.9611, 214.4762) construction
  line L8352 (206.9611, 214.4762) -> (207.0023, 214.6301) construction
  line L8353 (207.0023, 214.6301) -> (207.0447, 214.7839) construction
  line L8354 (207.0447, 214.7839) -> (207.0881, 214.9376) construction
  line L8355 (207.0881, 214.9376) -> (207.1327, 215.0912) construction
  line L8356 (207.1327, 215.0912) -> (207.1784, 215.2447) construction
  line L8357 (207.1784, 215.2447) -> (207.2252, 215.398) construction
  line L8358 (207.2252, 215.398) -> (207.2731, 215.5513) construction
  line L8359 (207.2731, 215.5513) -> (207.3221, 215.7044) construction
  line L8360 (207.3221, 215.7044) -> (207.3721, 215.8574) construction
  line L8361 (207.3721, 215.8574) -> (207.4233, 216.0103) construction
  line L8362 (207.4233, 216.0103) -> (207.4754, 216.1631) construction
  line L8363 (207.4754, 216.1631) -> (207.5285, 216.3158) construction
  line L8364 (207.5285, 216.3158) -> (207.5827, 216.4683) construction
  line L8365 (207.5827, 216.4683) -> (207.6378, 216.6206) construction
  line L8366 (207.6378, 216.6206) -> (207.694, 216.7729) construction
  line L8367 (207.694, 216.7729) -> (207.751, 216.925) construction
  line L8368 (207.751, 216.925) -> (207.8091, 217.077) construction
  line L8369 (207.8091, 217.077) -> (207.8681, 217.2288) construction
  line L8370 (207.8681, 217.2288) -> (207.9281, 217.3804) construction
  line L8371 (207.9281, 217.3804) -> (207.989, 217.532) construction
  line L8372 (207.989, 217.532) -> (208.0508, 217.6833) construction
  line L8373 (208.0508, 217.6833) -> (208.1135, 217.8345) construction
  line L8374 (208.1135, 217.8345) -> (208.1772, 217.9856) construction
  line L8375 (208.1772, 217.9856) -> (208.2417, 218.1365) construction
  line L8376 (208.2417, 218.1365) -> (208.3071, 218.2872) construction
  line L8377 (208.3071, 218.2872) -> (208.3735, 218.4378) construction
  line L8378 (208.3735, 218.4378) -> (208.4407, 218.5882) construction
  line L8379 (208.4407, 218.5882) -> (208.5087, 218.7384) construction
  line L8380 (208.5087, 218.7384) -> (208.5777, 218.8885) construction
  line L8381 (208.5777, 218.8885) -> (208.6474, 219.0384) construction
  line L8382 (208.6474, 219.0384) -> (208.7181, 219.1881) construction
  line L8383 (208.7181, 219.1881) -> (208.7895, 219.3376) construction
  line L8384 (208.7895, 219.3376) -> (208.8619, 219.487) construction
  line L8385 (208.8619, 219.487) -> (208.935, 219.6362) construction
  line L8386 (208.935, 219.6362) -> (209.009, 219.7852) construction
  line L8387 (209.009, 219.7852) -> (209.0838, 219.934) construction
  line L8388 (209.0838, 219.934) -> (209.1594, 220.0826) construction
  line L8389 (209.1594, 220.0826) -> (209.2358, 220.2311) construction
  line L8390 (209.2358, 220.2311) -> (209.313, 220.3793) construction
  line L8391 (209.313, 220.3793) -> (209.391, 220.5274) construction
  line L8392 (209.391, 220.5274) -> (209.4698, 220.6752) construction
  line L8393 (209.4698, 220.6752) -> (209.5494, 220.8229) construction
  line L8394 (209.5494, 220.8229) -> (209.6297, 220.9703) construction
  line L8395 (209.6297, 220.9703) -> (209.7109, 221.1176) construction
  line L8396 (209.7109, 221.1176) -> (209.7764, 221.2352) construction
  line L8397 (209.7764, 221.2352) -> (209.8259, 221.3234) construction
  line L8398 (209.8259, 221.3234) -> (209.8591, 221.3821) construction
  line L8399 (209.8591, 221.3821) -> (209.8757, 221.4115) construction